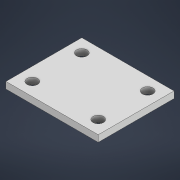
# Autodesk Inventor part: Ebene3_verbindung
Saved by Autodesk Inventor 2021 (Build 250183000, 183)
## iProperties
Created: 2021-02-07
Part Number: Ebene3_verbindung
Material: Generisch
Document SubType Name: Modeling
Designer: laure
Density: 1 g/cm^3
Appearance: Vorgabe
Author: laure
Autodesk Inventor part; units mm, degrees
ref_plane "YZ Plane" through (0, 0, 0) normal (1, 0, 0) x (0, 1, 0)
ref_plane "XZ Plane" through (0, 0, 0) normal (0, 1, 0) x (-1, 0, 0)
ref_plane "XY Plane" through (0, 0, 0) normal (0, 0, 1) x (1, 0, 0)
sketch "Skizze1" plane through (0, 0, 0) normal (0, 1, 0) x (-1, 0, 0)
  line L0 (14, -11.5) -> (-14, -11.5)
  line L1 (-14, -11.5) -> (-14, 11.5)
  line L2 (-14, 11.5) -> (14, 11.5)
  line L3 (14, 11.5) -> (14, -11.5)
  line L4 (0, -16.1) -> (0, 16.1) projected
  line L5 (-19.6, 0) -> (19.6, 0) projected
  point P0 (0, 0)
  dimension "d0" = 28
  dimension "d1" = 23
  constraints: 8 end point, 2 parallel, 1 horizontal, 1 perpendicular, 2 other
  measures "d0" distance between parallel lines of L1 L3
  measures "d1" distance between parallel lines of L2 L0
extrude "Extrusion1" add sketch "Skizze1" along normal mid plane 2
sketch "Skizze2" plane through (0, 1, 0) normal (0, 1, 0) x (1, 0, 0)
  circle A0 centre (-10, 7.5) radius 1.6
  circle A1 centre (-10, -7.5) radius 1.6
  circle A2 centre (10, 7.5) radius 1.6
  circle A3 centre (10, -7.5) radius 1.6
  line L0 (0, 16.1) -> (0, -16.1) projected
  line L1 (19.6, 0) -> (-19.6, 0) projected
  point P0 (0, 0)
  dimension "d4" = 3.2
  dimension "d5" = 3.2
  dimension "d6" = 3.2
  dimension "d7" = 3.2
  dimension "d8" = 20
  dimension "d9" = 20
  dimension "d10" = 15
  dimension "d11" = 15
  dimension "d12" = 7.5
  dimension "d13" = 10
  dimension "d14" = 10
  dimension "d15" = 7.5
  constraints: 4 centre point
  measures "d4" diameter of A0
  measures "d5" diameter of A1
  measures "d6" diameter of A2
  measures "d7" diameter of A3
  measures "d8" distance of A2.centre A0.centre
  measures "d9" distance of A3.centre A1.centre
  measures "d10" distance of A1.centre A0.centre
  measures "d11" distance of A3.centre A2.centre
  measures "d12" distance from line of L1 A1.centre
  measures "d13" distance from line of L0 A1.centre
  measures "d14" distance from line of L0 A0.centre
  measures "d15" distance from line of L1 A3.centre
extrude "Extrusion2" cut sketch "Skizze2" against normal up to surface (2 mm away)
